Autodesk Inventor part; units mm, degrees
(part 3 of 3)
  spline S676 degree 2 poles (-31.1598, 75.3019) (-31.1598, 75.2377) (-31.1781, 75.1827) knots 0 0 0 1 1 1
  line L434 (-31.1781, 75.1827) -> (-32.8372, 70.8059)
  spline S677 degree 2 poles (-32.8372, 70.8059) (-32.9793, 70.5905) (-33.1901, 70.5905) knots 0 0 0 1 1 1
  spline S678 degree 2 poles (-33.1901, 70.5905) (-33.4009, 70.5905) (-33.5476, 70.8014) knots 0 0 0 1 1 1
  line L435 (-33.5476, 70.8014) -> (-35.2799, 75.1644)
  line L436 (-34.1067, 74.0324) -> (-33.1992, 71.6446)
  line L437 (-33.1992, 71.6446) -> (-32.3193, 74.0324)
  line L438 (-32.3193, 74.0324) -> (-34.1067, 74.0324)
  spline S679 degree 2 poles (-39.8217, 75.2881) (-39.8217, 75.641) (-39.5147, 75.641) knots 0 0 0 1 1 1
  spline S680 degree 2 poles (-39.5147, 75.641) (-39.313, 75.641) (-39.1801, 75.4485) knots 0 0 0 1 1 1
  line L439 (-39.1801, 75.4485) -> (-36.8336, 71.8554)
  line L440 (-36.8336, 71.8554) -> (-36.8336, 75.279)
  spline S681 degree 2 poles (-36.8336, 75.279) (-36.8336, 75.641) (-36.4853, 75.641) knots 0 0 0 1 1 1
  spline S682 degree 2 poles (-36.4853, 75.641) (-36.137, 75.641) (-36.137, 75.279) knots 0 0 0 1 1 1
  line L441 (-36.137, 75.279) -> (-36.137, 70.9526)
  spline S683 degree 2 poles (-36.137, 70.9526) (-36.137, 70.6089) (-36.4669, 70.6089) knots 0 0 0 1 1 1
  spline S684 degree 2 poles (-36.4669, 70.6089) (-36.6869, 70.6089) (-36.8473, 70.8472) knots 0 0 0 1 1 1
  line L442 (-36.8473, 70.8472) -> (-39.1251, 74.3486)
  line L443 (-39.1251, 74.3486) -> (-39.1251, 70.9709)
  spline S685 degree 2 poles (-39.1251, 70.9709) (-39.1251, 70.6089) (-39.4734, 70.6089) knots 0 0 0 1 1 1
  spline S686 degree 2 poles (-39.4734, 70.6089) (-39.8217, 70.6089) (-39.8217, 70.9709) knots 0 0 0 1 1 1
  line L444 (-39.8217, 70.9709) -> (-39.8217, 75.2881)
  line L445 (-48.3507, 70.3018) -> (-46.7833, 70.3018)
  line L446 (-46.7833, 70.3018) -> (-46.7833, 75.4256)
  spline S687 degree 2 poles (-46.7833, 75.4256) (-46.7833, 75.7877) (-46.4167, 75.7877) knots 0 0 0 1 1 1
  spline S688 degree 2 poles (-46.4167, 75.7877) (-46.0546, 75.7877) (-46.0546, 75.4256) knots 0 0 0 1 1 1
  line L447 (-46.0546, 75.4256) -> (-46.0546, 70.3018)
  line L448 (-46.0546, 70.3018) -> (-44.4826, 70.3018)
  spline S689 degree 2 poles (-44.4826, 70.3018) (-44.1206, 70.3018) (-44.1206, 69.9306) knots 0 0 0 1 1 1
  spline S690 degree 2 poles (-44.1206, 69.9306) (-44.1206, 69.5685) (-44.4826, 69.5685) knots 0 0 0 1 1 1
  line L449 (-44.4826, 69.5685) -> (-48.3507, 69.5685)
  spline S691 degree 2 poles (-48.3507, 69.5685) (-48.7174, 69.5685) (-48.7174, 69.9306) knots 0 0 0 1 1 1
  spline S692 degree 2 poles (-48.7174, 69.9306) (-48.7174, 70.3018) (-48.3507, 70.3018) knots 0 0 0 1 1 1
  spline S693 degree 2 poles (-53.3966, 73.1387) (-53.3966, 74.1103) (-52.9062, 74.839) knots 0 0 0 1 1 1
  spline S694 degree 2 poles (-52.9062, 74.839) (-52.3654, 75.641) (-51.5176, 75.641) knots 0 0 0 1 1 1
  spline S695 degree 2 poles (-51.5176, 75.641) (-50.6697, 75.641) (-50.1289, 74.8298) knots 0 0 0 1 1 1
  spline S696 degree 2 poles (-50.1289, 74.8298) (-49.6431, 74.1011) (-49.6431, 73.1387) knots 0 0 0 1 1 1
  spline S697 degree 2 poles (-49.6431, 73.1387) (-49.6431, 72.1808) (-50.1243, 71.4705) knots 0 0 0 1 1 1
  spline S698 degree 2 poles (-50.1243, 71.4705) (-50.6881, 70.6501) (-51.5176, 70.6501) knots 0 0 0 1 1 1
  spline S699 degree 2 poles (-51.5176, 70.6501) (-52.4021, 70.6501) (-52.8742, 71.4155) knots 0 0 0 1 1 1
  spline S700 degree 2 poles (-52.8742, 71.4155) (-53.3966, 72.1671) (-53.3966, 73.1387) knots 0 0 0 1 1 1
  spline S701 degree 2 poles (-52.7, 73.1387) (-52.7, 72.4237) (-52.4342, 71.9654) knots 0 0 0 1 1 1
  spline S702 degree 2 poles (-52.4342, 71.9654) (-52.0905, 71.3559) (-51.5176, 71.3559) knots 0 0 0 1 1 1
  spline S703 degree 2 poles (-51.5176, 71.3559) (-50.9814, 71.3559) (-50.6422, 71.9242) knots 0 0 0 1 1 1
  spline S704 degree 2 poles (-50.6422, 71.9242) (-50.3397, 72.4375) (-50.3397, 73.1387) knots 0 0 0 1 1 1
  spline S705 degree 2 poles (-50.3397, 73.1387) (-50.3397, 73.8582) (-50.4956, 74.3257) knots 0 0 0 1 1 1
  spline S706 degree 2 poles (-50.4956, 74.3257) (-50.963, 74.9352) (-51.5176, 74.9352) knots 0 0 0 1 1 1
  spline S707 degree 2 poles (-51.5176, 74.9352) (-52.0767, 74.9352) (-52.5442, 74.3257) knots 0 0 0 1 1 1
  spline S708 degree 2 poles (-52.5442, 74.3257) (-52.7, 73.8536) (-52.7, 73.1387) knots 0 0 0 1 1 1
  spline S709 degree 2 poles (-57.8101, 72.0525) (-57.8101, 72.8087) (-57.338, 73.157) knots 0 0 0 1 1 1
  spline S710 degree 2 poles (-57.338, 73.157) (-56.9622, 73.4641) (-56.6185, 73.4641) knots 0 0 0 1 1 1
  line L450 (-56.6185, 73.4641) -> (-56.5772, 73.4595)
  line L451 (-56.5772, 73.4595) -> (-57.7413, 75.0773)
  spline S711 degree 2 poles (-57.7413, 75.0773) (-57.8101, 75.1873) (-57.8101, 75.2881) knots 0 0 0 1 1 1
  spline S712 degree 2 poles (-57.8101, 75.2881) (-57.8101, 75.4348) (-57.5947, 75.6502) (-57.4526, 75.6502) knots 0 0 0 1 2 2 2
  spline S713 degree 2 poles (-57.4526, 75.6502) (-57.2876, 75.6502) (-57.2464, 75.5402) knots 0 0 0 1 1 1
  line L452 (-57.2464, 75.5402) -> (-55.7981, 73.4641)
  line L453 (-55.7981, 73.4641) -> (-54.9503, 73.4641)
  line L454 (-54.9503, 73.4641) -> (-54.9503, 75.2881)
  spline S714 degree 2 poles (-54.9503, 75.2881) (-54.9503, 75.6502) (-54.602, 75.6502) knots 0 0 0 1 1 1
  spline S715 degree 2 poles (-54.602, 75.6502) (-54.2536, 75.6502) (-54.2536, 75.2881) knots 0 0 0 1 1 1
  line L455 (-54.2536, 75.2881) -> (-54.2536, 70.6364)
  line L456 (-54.2536, 70.6364) -> (-56.3618, 70.6364)
  spline S716 degree 2 poles (-56.3618, 70.6364) (-56.9622, 70.6364) (-57.3655, 70.9938) knots 0 0 0 1 1 1
  spline S717 degree 2 poles (-57.3655, 70.9938) (-57.8101, 71.3926) (-57.8101, 72.0525) knots 0 0 0 1 1 1
  spline S718 degree 2 poles (-57.1134, 72.0525) (-57.1134, 71.7088) (-56.6781, 71.3421) (-56.3618, 71.3421) knots 0 0 0 1 2 2 2
  line L457 (-56.3618, 71.3421) -> (-54.9503, 71.3421)
  line L458 (-54.9503, 71.3421) -> (-54.9503, 72.7583)
  line L459 (-54.9503, 72.7583) -> (-56.6185, 72.7583)
  spline S719 degree 2 poles (-56.6185, 72.7583) (-56.7468, 72.7583) (-56.9072, 72.6116) knots 0 0 0 1 1 1
  spline S720 degree 2 poles (-56.9072, 72.6116) (-57.1134, 72.4192) (-57.1134, 72.0525) knots 0 0 0 1 1 1
  spline S721 degree 2 poles (-62.141, 72.0525) (-62.141, 72.8087) (-61.669, 73.157) knots 0 0 0 1 1 1
  spline S722 degree 2 poles (-61.669, 73.157) (-61.2932, 73.4641) (-60.9494, 73.4641) knots 0 0 0 1 1 1
  line L460 (-60.9494, 73.4641) -> (-60.9082, 73.4595)
  line L461 (-60.9082, 73.4595) -> (-62.0723, 75.0773)
  spline S723 degree 2 poles (-62.0723, 75.0773) (-62.141, 75.1873) (-62.141, 75.2881) knots 0 0 0 1 1 1
  spline S724 degree 2 poles (-62.141, 75.2881) (-62.141, 75.4348) (-61.9256, 75.6502) (-61.7835, 75.6502) knots 0 0 0 1 2 2 2
  spline S725 degree 2 poles (-61.7835, 75.6502) (-61.6186, 75.6502) (-61.5773, 75.5402) knots 0 0 0 1 1 1
  line L462 (-61.5773, 75.5402) -> (-60.1291, 73.4641)
  line L463 (-60.1291, 73.4641) -> (-59.2812, 73.4641)
  line L464 (-59.2812, 73.4641) -> (-59.2812, 75.2881)
  spline S726 degree 2 poles (-59.2812, 75.2881) (-59.2812, 75.6502) (-58.9329, 75.6502) knots 0 0 0 1 1 1
  spline S727 degree 2 poles (-58.9329, 75.6502) (-58.5846, 75.6502) (-58.5846, 75.2881) knots 0 0 0 1 1 1
  line L465 (-58.5846, 75.2881) -> (-58.5846, 70.6364)
  line L466 (-58.5846, 70.6364) -> (-60.6928, 70.6364)
  spline S728 degree 2 poles (-60.6928, 70.6364) (-61.2932, 70.6364) (-61.6965, 70.9938) knots 0 0 0 1 1 1
  spline S729 degree 2 poles (-61.6965, 70.9938) (-62.141, 71.3926) (-62.141, 72.0525) knots 0 0 0 1 1 1
  spline S730 degree 2 poles (-61.4444, 72.0525) (-61.4444, 71.7088) (-61.009, 71.3421) (-60.6928, 71.3421) knots 0 0 0 1 2 2 2
  line L467 (-60.6928, 71.3421) -> (-59.2812, 71.3421)
  line L468 (-59.2812, 71.3421) -> (-59.2812, 72.7583)
  line L469 (-59.2812, 72.7583) -> (-60.9494, 72.7583)
  spline S731 degree 2 poles (-60.9494, 72.7583) (-61.0778, 72.7583) (-61.2382, 72.6116) knots 0 0 0 1 1 1
  spline S732 degree 2 poles (-61.2382, 72.6116) (-61.4444, 72.4192) (-61.4444, 72.0525) knots 0 0 0 1 1 1
  line L470 (-65.9037, 75.5723) -> (-62.9201, 75.5723)
  line L471 (-62.9201, 75.5723) -> (-62.9201, 70.6364)
  line L472 (-62.9201, 70.6364) -> (-65.9037, 70.6364)
  spline S733 degree 2 poles (-65.9037, 70.6364) (-66.2612, 70.6364) (-66.2612, 70.9801) knots 0 0 0 1 1 1
  spline S734 degree 2 poles (-66.2612, 70.9801) (-66.2612, 71.333) (-65.9037, 71.333) knots 0 0 0 1 1 1
  line L473 (-65.9037, 71.333) -> (-63.6168, 71.333)
  line L474 (-63.6168, 71.333) -> (-63.6168, 72.4925)
  line L475 (-63.6168, 72.4925) -> (-65.7662, 72.4925)
  spline S735 degree 2 poles (-65.7662, 72.4925) (-66.1145, 72.4925) (-66.1145, 72.8454) knots 0 0 0 1 1 1
  spline S736 degree 2 poles (-66.1145, 72.8454) (-66.1145, 73.1983) (-65.7662, 73.1983) knots 0 0 0 1 1 1
  line L476 (-65.7662, 73.1983) -> (-63.6168, 73.1983)
  line L477 (-63.6168, 73.1983) -> (-63.6168, 74.8665)
  line L478 (-63.6168, 74.8665) -> (-65.9037, 74.8665)
  spline S737 degree 2 poles (-65.9037, 74.8665) (-66.2612, 74.8665) (-66.2612, 75.2194) knots 0 0 0 1 1 1
  spline S738 degree 2 poles (-66.2612, 75.2194) (-66.2612, 75.5723) (-65.9037, 75.5723) knots 0 0 0 1 1 1
  spline S739 degree 2 poles (-70.4913, 74.2294) (-70.4913, 75.6685) (-68.6902, 75.6685) knots 0 0 0 1 1 1
  spline S740 degree 2 poles (-68.6902, 75.6685) (-67.6406, 75.6685) (-67.0494, 74.6007) knots 0 0 0 1 1 1
  spline S741 degree 2 poles (-67.0494, 74.6007) (-67.0036, 74.5228) (-67.0036, 74.4265) knots 0 0 0 1 1 1
  spline S742 degree 2 poles (-67.0036, 74.4265) (-67.0036, 74.2707) (-67.2328, 74.0415) (-67.384, 74.0415) knots 0 0 0 1 2 2 2
  spline S743 degree 2 poles (-67.384, 74.0415) (-67.5627, 74.0415) (-67.6452, 74.2203) knots 0 0 0 1 1 1
  spline S744 degree 2 poles (-67.6452, 74.2203) (-67.9844, 74.9719) (-68.6902, 74.9719) knots 0 0 0 1 1 1
  spline S745 degree 2 poles (-68.6902, 74.9719) (-69.7901, 74.9719) (-69.7901, 74.2432) knots 0 0 0 1 1 1
  spline S746 degree 2 poles (-69.7901, 74.2432) (-69.7901, 73.8536) (-69.1714, 73.5695) knots 0 0 0 1 1 1
  spline S747 degree 2 poles (-69.1714, 73.5695) (-68.4335, 73.2716) (-67.8102, 73.0195) knots 0 0 0 1 1 1
  spline S748 degree 2 poles (-67.8102, 73.0195) (-67.054, 72.5887) (-67.054, 71.8738) knots 0 0 0 1 1 1
  spline S749 degree 2 poles (-67.054, 71.8738) (-67.054, 70.6043) (-68.6077, 70.5401) knots 0 0 0 1 1 1
  spline S750 degree 2 poles (-68.6077, 70.5401) (-69.2035, 70.5126) (-70.1246, 71.0626) (-70.3034, 71.6034) knots 0 0 0 1 2 2 2
  spline S751 degree 2 poles (-70.3034, 71.6034) (-70.3309, 71.663) (-70.3309, 71.718) knots 0 0 0 1 1 1
  spline S752 degree 2 poles (-70.3309, 71.718) (-70.3309, 72.0388) (-69.9688, 72.0388) knots 0 0 0 1 1 1
  spline S753 degree 2 poles (-69.9688, 72.0388) (-69.7168, 72.0388) (-69.6388, 71.8004) knots 0 0 0 1 1 1
  spline S754 degree 2 poles (-69.6388, 71.8004) (-69.5472, 71.5301) (-68.9835, 71.2184) (-68.6397, 71.2367) knots 0 0 0 1 2 2 2
  spline S755 degree 2 poles (-68.6397, 71.2367) (-67.7644, 71.278) (-67.7644, 71.8554) knots 0 0 0 1 1 1
  spline S756 degree 2 poles (-67.7644, 71.8554) (-67.7644, 72.2633) (-68.3739, 72.5337) knots 0 0 0 1 1 1
  spline S757 degree 2 poles (-68.3739, 72.5337) (-69.1255, 72.85) (-69.7351, 73.0791) knots 0 0 0 1 1 1
  spline S758 degree 2 poles (-69.7351, 73.0791) (-70.4913, 73.5007) (-70.4913, 74.2294) knots 0 0 0 1 1 1
  dimension "d123" = 10
  dimension "d124" = 80
  dimension "d125" = 60
  dimension "d126" = 100
  dimension "d127" = 25
  constraints: 2 other
  measures "d123" distance between parallel lines of L4 L3
  measures "d124" distance between parallel lines of L3 L1
  measures "d125" distance between parallel lines of L0 L2
  measures "d126" distance between parallel lines of L5 L4
  measures "d127" distance between parallel lines of L6 L0
extrude "Extrusion14" cut sketch "Sketch13" against normal blind 1
equation "\"d103\" = d101"
equation "\"d88\" = d86"
equation "\"d123\" = -0.5 * d124 + 0.5 * d126"
equation "\"d86\" = 5"
body "Solid1"
